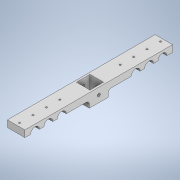
# Autodesk Inventor part: holder
Saved by Autodesk Inventor 2020 (Build 240168000, 168)
## iProperties
Created: 2020-04-27
Part Number: holder
Material: Generic
Document SubType Name: Modeling
Designer: Clevo
Density: 1 g/cm^3
Appearance: Default
Author: Clevo
Autodesk Inventor part; units mm, degrees
ref_plane "YZ Plane" through (0, 0, 0) normal (1, 0, 0) x (0, 1, 0)
ref_plane "XZ Plane" through (0, 0, 0) normal (0, 1, 0) x (-1, 0, 0)
ref_plane "XY Plane" through (0, 0, 0) normal (0, 0, 1) x (1, 0, 0)
sketch "Sketch1" plane through (0, 0, 0) normal (0, 1, 0) x (-1, 0, 0)
  line L0 (-13, -110) -> (13, -110)
  line L1 (13, -110) -> (13, 110)
  line L2 (13, 110) -> (-13, 110)
  line L3 (-13, 110) -> (-13, -110)
  line L4 (-13, -110) -> (13, 110) construction
  line L5 (13, -110) -> (-13, 110) construction
  point P0 (0, 0)
  dimension "d0" = 220
  dimension "d1" = 26
  constraints: 12 end point, 2 midpoint, 2 parallel, 1 horizontal, 1 perpendicular
  measures "d0" distance of L0.end L1.end
  measures "d1" distance of L0.start L0.end
extrude "Extrusion1" add sketch "Sketch1" along normal blind 10
sketch "Sketch3" plane through (0, 0, 0) normal (0, -1, 0) x (1, 0, 0)
  line L0 (13, 110) -> (13, -110) projected
  line L1 (-13, -14) -> (13, -14)
  line L2 (13, -14) -> (13, 14)
  line L3 (13, 14) -> (-13, 14)
  line L4 (-13, 14) -> (-13, -14)
  line L5 (-13, -14) -> (13, 14) construction
  line L6 (13, -14) -> (-13, 14) construction
  point P0 (0, 0)
  dimension "d4" = 28
  constraints: 12 end point, 2 midpoint, 2 parallel, 1 horizontal, 1 perpendicular, 1 point on line
  measures "d4" distance of L3.end L1.start
extrude "Extrusion2" add sketch "Sketch3" along normal blind 10
sketch "Sketch4" plane through (0, -10, 0) normal (0, -1, 0) x (1, 0, 0)
  line L0 (-10.125, 10.125) -> (10.125, 10.125)
  line L1 (10.125, 10.125) -> (10.125, -10.125)
  line L2 (10.125, -10.125) -> (-10.125, -10.125)
  line L3 (-10.125, -10.125) -> (-10.125, 10.125)
  line L4 (-10.125, 10.125) -> (10.125, -10.125) construction
  line L5 (10.125, 10.125) -> (-10.125, -10.125) construction
  point P0 (0, 0)
  dimension "d7" = 20.25
  dimension "d8" = 20.25
  constraints: 12 end point, 2 midpoint, 2 parallel, 1 horizontal, 1 perpendicular
  measures "d7" distance of L1.end L2.end
  measures "d8" distance of L0.end L1.end
extrude "Extrusion3" cut sketch "Sketch4" against normal through all
sketch "Sketch5" plane through (-13, 0, 110) normal (-1, 0, 0) x (0, 0, 1)
  point P0 (-110, 0)
hole "Hole1" at (-13, 0, 0) direction (1, 0, 0) diameter 4.3 end through all clearance for "Flat Head Machine Screw" size "M4" standard "Ansi Metric M Profile"
sketch "Sketch6" plane through (-13, 0, 110) normal (-1, 0, 0) x (0, 0, 1)
  circle A0 centre (-35, 0) radius 6.6
  line L0 (-96, 0) -> (0, 0) projected
  point P0 (-110, 0)
  dimension "d18" = 75
  dimension "d19" = 13.2
  constraints: 1 centre point, 1 point on line
  measures "d18" distance of point (-110, 0) A0.centre
  measures "d19" diameter of A0
extrude "Extrusion4" cut sketch "Sketch6" against normal through all
sketch "Sketch7" plane through (0, 0, 0) normal (0, -1, 0) x (1, 0, 0)
  line L0 (-13, 81.6) -> (13, 81.6) projected
  line L1 (-13, 68.4) -> (-13, 81.6) projected
  line L2 (13, 68.4) -> (-13, 68.4) projected
  line L3 (13, 81.6) -> (13, 68.4) projected
  line L4 (0, 85) -> (0, 65)
  point P0 (0, 0)
  point P1 (0, 75)
  point P2 (13, 75)
  point P3 (0, 68.4)
  dimension "d22" = 20
  constraints: 3 midpoint, 2 end point, 1 horizontal alignment, 1 vertical, 1 vertical alignment
  measures "d22" distance of L4.start L4.end
hole "Hole2" at (0, 0, 65) at (0, 0, 85) direction (0, 1, 0) diameter 2.459 end through all thread size "M3x0.5" class "6H" standard "ANSI Metric M Profile"
pattern_linear "Rectangular Pattern1" count 2 spacing 20 along (0, 0, 1) count 2 spacing 20 along (0, 0, -1) of "Extrusion4"
pattern_linear "Rectangular Pattern2" count 2 spacing 20 along (0, 0, 1) count 2 spacing 20 along (0, 0, -1) of "Hole2"
mirror "Mirror1" about plane through (0, 0, 0) normal (0, 0, 1) of "Extrusion4", "Hole2", "Rectangular Pattern1", "Rectangular Pattern2"
fillet "Fillet1" radius 5 2 edges at (0, 0, 14) (0, 0, -14)
body "Solid1"
